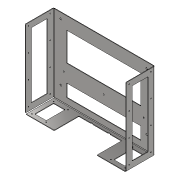
# Autodesk Inventor part: Display_Mount_B
Saved by Autodesk Inventor 2020 (Build 240168000, 168)
## iProperties
Created: 2021-12-05
Part Number: Display_Mount_B
Material: ステンレス鋼
Document SubType Name: Sheet Metal
Designer: ken113
Density: 8 g/cm^3
Sheet Metal Rule: Default_mm
Appearance: 半つや出し
Mass: 1681.3 g
Surface Area: 2199.78 cm^2
Volume: 210.162 cm^3
Author: ken113
Autodesk Inventor part; units mm, degrees
ref_plane "YZ Plane" through (0, 0, 0) normal (1, 0, 0) x (0, 1, 0)
ref_plane "XZ Plane" through (0, 0, 0) normal (0, 1, 0) x (-1, 0, 0)
ref_plane "XY Plane" through (0, 0, 0) normal (0, 0, 1) x (1, 0, 0)
sketch "スケッチ1" plane through (0, 0, 0) normal (0, 0, 1) x (1, 0, 0)
  line L0 (173, -134) -> (-173, -134)
  line L1 (-173, -134) -> (-173, 134)
  line L2 (-173, 134) -> (173, 134)
  line L3 (173, 134) -> (173, -134)
  line L4 (173, -134) -> (-173, 134) construction
  line L5 (-173, -134) -> (173, 134) construction
  point P0 (0, 0)
  dimension "d0" = 268
  dimension "d1" = 346
  measures "d0" distance of L0.end L1.end
  measures "d1" distance of L1.end L2.end
extrude "プレート1" add sketch "スケッチ1" along normal blind 2
sketch "スケッチ2" plane through (173, -136, 4) normal (0, -1, 0) x (1, 0, 0)
  line L0 (-346, 0) -> (0, 0)
  line L1 (0, 0) -> (0, 96)
  line L2 (0, 96) -> (-346, 96)
  line L3 (-346, 96) -> (-346, 0)
  constraints: 6 end point, 1 horizontal, 1 perpendicular, 1 vertical
edge flange "フランジ1" height 100 angle 90 thickness 2 bend radius 2 thickness toward (0, -1, 0) relief straight relief width 2 relief depth 1 edges at (0, -134, 2) wall of the first edge with corners at (-173, -136, 4) (173, -136, 4) (173, -136, 100) (-173, -136, 100)
bend "曲げ1"
corner "コーナー1"
sketch "スケッチ3" plane through (0, 0, 2) normal (0, 0, 1) x (1, 0, 0)
  line L0 (150, -86) -> (-150, -86)
  line L1 (-150, -86) -> (-150, 114)
  line L2 (-150, 114) -> (150, 114)
  line L3 (150, 114) -> (150, -86)
  line L4 (150, -86) -> (-150, 114) construction
  line L5 (-150, -86) -> (150, 114) construction
  line L6 (173, -134) -> (-173, -134) projected
  line L7 (-173, 134) -> (173, 134) projected
  point P0 (0, 0)
  point P1 (0, 14)
  point P2 (0, 14)
  dimension "d13" = 300
  dimension "d14" = 200
  dimension "d51" = 120
  constraints: 12 end point, 3 midpoint, 2 parallel, 1 horizontal, 1 perpendicular, 1 vertical alignment
  measures "d13" distance of L0.start L0.end
  measures "d14" distance of L0.end L1.end
  measures "d51" distance from line of L7 point (0, 14)
hole "穴1" at (-150, 114, 2) at (-150, -86, 2) at (150, -86, 2) at (150, 114, 2) direction (0, 0, -1) diameter 6.2 depth 2 tip angle 118
sketch "スケッチ4" plane through (0, 0, 2) normal (0, 0, 1) x (1, 0, 0)
  line L0 (130, -9.8) -> (-130, -9.8)
  line L1 (-130, -9.8) -> (-130, 90.2)
  line L2 (-130, 90.2) -> (130, 90.2)
  line L3 (130, 90.2) -> (130, -9.8)
  line L4 (130, -9.8) -> (-130, 90.2) construction
  line L5 (-130, -9.8) -> (130, 90.2) construction
  circle A0 centre (-150, 114) radius 3.1 projected
  point P0 (0, 0)
  point P1 (0, 40.2)
  point P2 (0, 40.2)
  dimension "d23" = 100
  dimension "d24" = 23.8
  dimension "d25" = 260
  constraints: 12 end point, 3 midpoint, 2 parallel, 1 horizontal, 1 perpendicular, 1 vertical alignment
  measures "d23" distance of L2.end L0.start
  measures "d24" distance from line of L2 A0.centre
  measures "d25" distance of L1.end L2.end
extrude "押し出し1" cut sketch "スケッチ4" against normal through all contours L0 L1 L2 L3
fillet "フィレット1" radius 2 4 edges at (130, -9.8, 1) (130, 90.2, 1) (-130, 90.2, 1) (-130, -9.8, 1)
sketch "スケッチ6" plane through (175, 134, 4) normal (1, 0, 0) x (0, 1, 0)
  line L0 (-268, 0) -> (0, 0)
  line L1 (0, 0) -> (0, 96)
  line L2 (0, 96) -> (-268, 96)
  line L3 (-268, 96) -> (-268, 0)
  constraints: 6 end point, 1 horizontal, 1 perpendicular, 1 vertical
edge flange "フランジ2" height 100 angle 90 thickness 2 bend radius 2 thickness toward (1, 0, 0) relief straight relief width 2 relief depth 1 corner gap 2 corner form 0 edges at (173, 0, 2) (-173, 0, 2) wall of the first edge with corners at (175, -134, 4) (175, 134, 4) (175, 134, 100) (175, -134, 100)
bend "曲げ2"
corner "コーナー2"
fillet "フィレット2" radius 2 6 edges at (-176, 134, 100) (-176, -134, 100) (-173, -137, 100) (173, -137, 100) (176, -134, 100) (176, 134, 100)
sketch "スケッチ7" plane through (-177, -134, 4) normal (-1, 0, 0) x (0, 0, 1)
  arc A0 (94, 0) -> (96, 2) centre (94, 2) ccw projected
  line L0 (96, 266) -> (96, 2) projected
  arc A1 (96, 266) -> (94, 268) centre (94, 266) ccw projected
  line L1 (0, 268) -> (94, 268) projected
  line L2 (0, 268) -> (0, 0) projected
  line L3 (94, 0) -> (0, 0) projected
  line L4 (10, 258) -> (86, 258)
  line L5 (86, 258) -> (86, 14)
  line L6 (86, 14) -> (10, 14)
  line L7 (10, 14) -> (10, 258)
  line L8 (10, 95.3333) -> (86, 95.3333)
  line L9 (86, 95.3333) -> (86, 176.6667)
  line L10 (86, 176.6667) -> (10, 176.6667)
  line L11 (10, 176.6667) -> (10, 95.3333)
  point P0 (-4, 134)
  dimension "d52" = 10
  dimension "d53" = 10
  dimension "d54" = 10
  dimension "d55" = 14
  dimension "d56" = 244
  dimension "d57" = 81.3333
  dimension "d58" = 81.3333
  constraints: 16 end point, 4 parallel, 2 horizontal, 2 perpendicular, 2 point on line
  measures "d52" distance between parallel lines of L7 L2
  measures "d53" distance between parallel lines of L1 L4
  measures "d54" distance between parallel lines of L0 L5
  measures "d55" distance between parallel lines of L6 L3
  measures "d56" distance of L4.end L5.end
  measures "d57" distance between parallel lines of L4 L10
  measures "d58" distance between parallel lines of L10 L8
hole "穴3" at (-177, -120, 14) at (-177, -120, 90) at (-177, -38.6667, 90) at (-177, -38.6667, 14) at (-177, 42.6667, 14) at (-177, 42.6667, 90) at (-177, 124, 90) at (-177, 124, 14) direction (1, 0, 0) diameter 3.242 end through all thread size "M4x0.7" class "6H" standard "ISO Metric profile"
sketch "スケッチ8" plane through (-173, -138, 4) normal (0, -1, 0) x (1, 0, 0)
  arc A0 (346, 94) -> (344, 96) centre (344, 94) ccw projected
  line L0 (2, 96) -> (344, 96) projected
  arc A1 (2, 96) -> (0, 94) centre (2, 94) ccw projected
  line L1 (0, 0) -> (0, 94) projected
  line L2 (0, 0) -> (346, 0) projected
  line L3 (346, 94) -> (346, 0) projected
  line L4 (10, 86) -> (60, 86)
  line L5 (60, 86) -> (60, 10)
  line L6 (60, 10) -> (10, 10)
  line L7 (10, 10) -> (10, 86)
  line L8 (286, 10) -> (336, 10)
  line L9 (336, 10) -> (336, 86)
  line L10 (336, 86) -> (286, 86)
  line L11 (286, 86) -> (286, 10)
  point P0 (173, -4)
  dimension "d66" = 50
  dimension "d67" = 50
  dimension "d68" = 10
  dimension "d69" = 10
  dimension "d70" = 10
  dimension "d71" = 10
  constraints: 16 end point, 4 parallel, 2 horizontal, 2 horizontal alignment, 2 perpendicular, 1 point on line
  measures "d66" distance of L4.start L4.end
  measures "d67" distance of L9.end L10.end
  measures "d68" distance between parallel lines of L6 L2
  measures "d69" distance between parallel lines of L0 L10
  measures "d70" distance between parallel lines of L3 L9
  measures "d71" distance between parallel lines of L1 L7
hole "穴4" at (-163, -138, 14) at (-113, -138, 90) at (-113, -138, 14) at (-163, -138, 90) at (113, -138, 14) at (163, -138, 14) at (163, -138, 90) at (113, -138, 90) direction (0, 1, 0) diameter 3.242 end through all thread size "M4x0.7" class "6H" standard "ISO Metric profile"
sketch "スケッチ9" plane through (-177, -134, 4) normal (-1, 0, 0) x (0, 0, 1)
  circle A0 centre (86, 258) radius 1.621 projected
  circle A1 centre (10, 176.6667) radius 1.621 projected
  circle A2 centre (86, 95.3333) radius 1.621 projected
  circle A3 centre (10, 14) radius 1.621 projected
  circle A4 centre (86, 14) radius 1.621 projected
  circle A5 centre (10, 95.3333) radius 1.621 projected
  circle A6 centre (86, 176.6667) radius 1.621 projected
  circle A7 centre (10, 258) radius 1.621 projected
  arc A8 (94, 0) -> (96, 2) centre (94, 2) ccw projected
  line L0 (96, 266) -> (96, 2) projected
  arc A9 (96, 266) -> (94, 268) centre (94, 266) ccw projected
  line L1 (0, 268) -> (94, 268) projected
  line L2 (0, 268) -> (0, 0) projected
  line L3 (94, 0) -> (0, 0) projected
  line L4 (20, 248) -> (76, 248)
  line L5 (76, 248) -> (76, 20)
  line L6 (76, 20) -> (20, 20)
  line L7 (20, 20) -> (20, 248)
  point P0 (-4, 134)
  dimension "d79" = 20
  dimension "d80" = 20
  dimension "d81" = 20
  dimension "d82" = 20
  constraints: 8 end point, 2 parallel, 1 horizontal, 1 perpendicular
  measures "d79" distance between parallel lines of L0 L5
  measures "d80" distance between parallel lines of L2 L7
  measures "d81" distance between parallel lines of L1 L4
  measures "d82" distance between parallel lines of L3 L6
extrude "押し出し2" cut sketch "スケッチ9" against normal through all contours L4 L5 L6 L7
fillet "フィレット3" radius 2 8 edges at (-176, 114, 24) (-176, 114, 80) (-176, -114, 24) (-176, -114, 80) (176, -114, 24) (176, -114, 80) (176, 114, 80) (176, 114, 24)
sketch "スケッチ11" plane through (0, 0, 2) normal (0, 0, 1) x (1, 0, 0)
  line L0 (130, 88.2) -> (130, -7.8) projected
  arc A0 (128, -9.8) -> (130, -7.8) centre (128, -7.8) ccw projected
  line L1 (128, -9.8) -> (-128, -9.8) projected
  arc A1 (-130, -7.8) -> (-128, -9.8) centre (-128, -7.8) ccw projected
  line L2 (-130, -7.8) -> (-130, 88.2) projected
  arc A2 (-128, 90.2) -> (-130, 88.2) centre (-128, 88.2) ccw projected
  line L3 (-128, 90.2) -> (128, 90.2) projected
  arc A3 (130, 88.2) -> (128, 90.2) centre (128, 88.2) ccw projected
  circle A4 centre (150, -86) radius 3.1 projected
  circle A5 centre (-150, 114) radius 3.1 projected
  circle A6 centre (-150, -86) radius 3.1 projected
  circle A7 centre (150, 114) radius 3.1 projected
  line L4 (-173, -134) -> (-173, 134) projected
  line L5 (173, -134) -> (-173, -134) projected
  line L6 (173, 134) -> (173, -134) projected
  line L7 (-173, 134) -> (173, 134) projected
  point P0 (0, 0)
  point P1 (-140, -39.8)
  point P2 (0, -39.8)
  point P3 (140, -39.8)
  dimension "d89" = 140
  dimension "d94" = 30
  constraints: 1 horizontal, 1 vertical alignment, 2 other
  measures "d89" distance of point (-140, -39.8) point (0, -39.8)
  measures "d94" distance from line of L1 point (-140, -39.8)
hole "穴5" at (-140, -39.8, 2) at (0, -39.8, 2) at (140, -39.8, 2) direction (0, 0, -1) diameter 4.3 end through all
sketch "スケッチ12" plane through (0, 0, 0) normal (0, 0, -1) x (-1, 0, 0)
  circle A0 centre (0, -39.8) radius 2.15 projected
  circle A1 centre (140, -39.8) radius 2.15 projected
  circle A2 centre (-140, -39.8) radius 2.15 projected
  line L0 (-130, -7.8) -> (-130, 88.2) projected
  arc A3 (-128, 90.2) -> (-130, 88.2) centre (-128, 88.2) ccw projected
  line L1 (-128, 90.2) -> (128, 90.2) projected
  arc A4 (130, 88.2) -> (128, 90.2) centre (128, 88.2) ccw projected
  line L2 (130, 88.2) -> (130, -7.8) projected
  arc A5 (128, -9.8) -> (130, -7.8) centre (128, -7.8) ccw projected
  line L3 (128, -9.8) -> (-128, -9.8) projected
  arc A6 (-130, -7.8) -> (-128, -9.8) centre (-128, -7.8) ccw projected
  circle A7 centre (-150, -86) radius 3.1 projected
  circle A8 centre (150, 114) radius 3.1 projected
  circle A9 centre (150, -86) radius 3.1 projected
  circle A10 centre (-150, 114) radius 3.1 projected
  line L4 (-173, -134) -> (173, -134) projected
  line L5 (173, -134) -> (173, 134) projected
  line L6 (173, 134) -> (-173, 134) projected
  line L7 (-173, 134) -> (-173, -134) projected
  point P0 (0, 0)
hole "穴6" at (140, -39.8, 0) at (0, -39.8, 0) at (-140, -39.8, 0) direction (0, 0, 1) diameter 4.2 end through all countersink diameter 8 countersink angle 90
sketch "スケッチ13" plane through (0, 0, 2) normal (0, 0, 1) x (1, 0, 0)
  line L0 (-130, -114) -> (130, -114)
  line L1 (130, -114) -> (130, -69.8)
  line L2 (130, -69.8) -> (-130, -69.8)
  line L3 (-130, -69.8) -> (-130, -114)
  circle A0 centre (0, -39.8) radius 2.15 projected
  line L4 (173, -134) -> (-173, -134) projected
  point P0 (0, 0)
  point P1 (-130, 88.2)
  point P2 (130, -7.8)
  dimension "d109" = 30
  dimension "d110" = 20
  constraints: 8 end point, 2 parallel, 2 vertical alignment, 1 horizontal, 1 perpendicular
  measures "d109" distance from line of A0.centre L2
  measures "d110" distance between parallel lines of L0 L4
extrude "押し出し3" cut sketch "スケッチ13" against normal blind 10 contours L3 L2 L1 L0
fillet "フィレット4" radius 2 4 edges at (-130, -69.8, 1) (-130, -114, 1) (130, -114, 1) (130, -69.8, 1)
sketch "スケッチ14" plane through (-173, -136, 4) normal (0, 1, 0) x (1, 0, 0)
  line L0 (2, -96) -> (344, -96) projected
  line L1 (98, -96) -> (248, -96)
  line L2 (248, -96) -> (248, -10)
  line L3 (248, -10) -> (98, -10)
  line L4 (98, -10) -> (98, -96)
  line L5 (0, 2) -> (346, 2) projected
  line L6 (346, 0) -> (0, 0) projected
  point P0 (173, 4)
  point P1 (173, 4)
  dimension "d114" = 150
  dimension "d115" = 75
  dimension "d120" = 10
  constraints: 8 end point, 2 parallel, 1 coincident, 1 horizontal, 1 perpendicular, 1 point on line
  measures "d114" distance between parallel lines of L2 L4
  measures "d115" distance from line of L2 point (173, 4)
  measures "d120" distance between parallel lines of L3 L6
extrude "押し出し4" cut sketch "スケッチ14" against normal blind 10
fillet "フィレット5" radius 2 4 edges at (-75, -137, 100) (-75, -137, 14) (75, -137, 100) (75, -137, 14)
sketch "スケッチ15" plane through (-173, -138, 4) normal (0, -1, 0) x (1, 0, 0)
  line L0 (246, 10) -> (100, 10) projected
  point P0 (173, -4)
  point P1 (143, 14)
  point P2 (203, 14)
  dimension "d122" = 60
  dimension "d123" = 30
  dimension "d131" = 4
  constraints: 1 horizontal alignment
  measures "d122" distance of point (143, 14) point (203, 14)
  measures "d123" horizontal distance of point (203, 14) point (173, -4)
  measures "d131" distance from line of L0 point (143, 14)
hole "穴7" at (-30, -138, 18) at (30, -138, 18) direction (0, 1, 0) diameter 12 end through all
sketch "スケッチ16" plane through (-173, -136, 4) normal (0, 1, 0) x (1, 0, 0)
  arc A0 (147.4721, -10) -> (138.5279, -10) centre (143, -14) ccw projected
  line L0 (147.4721, -10) -> (198.5279, -10) projected
  arc A1 (207.4721, -10) -> (198.5279, -10) centre (203, -14) ccw projected
  line L1 (207.4721, -10) -> (246, -10) projected
  arc A2 (248, -12) -> (246, -10) centre (246, -12) ccw projected
  line L2 (248, -12) -> (248, -94) projected
  arc A3 (248, -94) -> (250, -96) centre (250, -94) ccw projected
  line L3 (250, -96) -> (344, -96) projected
  arc A4 (344, -96) -> (346, -94) centre (344, -94) ccw projected
  line L4 (346, -94) -> (346, 0) projected
  line L5 (346, 0) -> (0, 0) projected
  line L6 (0, -94) -> (0, 0) projected
  arc A5 (0, -94) -> (2, -96) centre (2, -94) ccw projected
  line L7 (2, -96) -> (96, -96) projected
  arc A6 (96, -96) -> (98, -94) centre (96, -94) ccw projected
  line L8 (98, -94) -> (98, -12) projected
  arc A7 (100, -10) -> (98, -12) centre (100, -12) ccw projected
  line L9 (100, -10) -> (138.5279, -10) projected
  circle A8 centre (336, -86) radius 1.621 projected
  circle A9 centre (286, -10) radius 1.621 projected
  circle A10 centre (60, -10) radius 1.621 projected
  circle A11 centre (10, -10) radius 1.621 projected
  circle A12 centre (60, -86) radius 1.621 projected
  circle A13 centre (10, -86) radius 1.621 projected
  circle A14 centre (336, -10) radius 1.621 projected
  circle A15 centre (286, -86) radius 1.621 projected
  circle A16 centre (10, -10) radius 1.621 projected
  circle A17 centre (60, -86) radius 1.621 projected
  line L10 (10, -10) -> (60, -10)
  line L11 (60, -10) -> (60, -86)
  line L12 (60, -86) -> (10, -86)
  line L13 (10, -86) -> (10, -10)
  circle A18 centre (286, -10) radius 1.621 projected
  circle A19 centre (336, -86) radius 1.621 projected
  line L14 (286, -10) -> (336, -10)
  line L15 (336, -10) -> (336, -86)
  line L16 (336, -86) -> (286, -86)
  line L17 (286, -86) -> (286, -10)
  line L18 (55, -15) -> (15, -15)
  line L19 (15, -15) -> (15, -81)
  line L20 (15, -81) -> (55, -81)
  line L21 (55, -81) -> (55, -15)
  line L22 (331, -15) -> (291, -15)
  line L23 (291, -15) -> (291, -81)
  line L24 (291, -81) -> (331, -81)
  line L25 (331, -81) -> (331, -15)
  point P0 (173, 4)
  dimension "d132" = 5
  dimension "d133" = 5
  constraints: 32 end point, 8 parallel, 4 perpendicular, 2 horizontal, 6 other
  measures "d132" distance between parallel lines of L11 L21
  measures "d133" distance between parallel lines of L17 L23
extrude "押し出し5" cut sketch "スケッチ16" against normal blind 10 contours L21 L20 L19 L18 | L25 L24 L23 L22
fillet "フィレット6" radius 2 8 edges at (-118, -137, 85) (-158, -137, 85) (-158, -137, 19) (-118, -137, 19) (118, -137, 85) (118, -137, 19) (158, -137, 85) (158, -137, 19)
equation "\"d21\" = Thickness"
equation "\"d57\" = 0.333333 * d56"
equation "\"d58\" = d57"
equation "\"d129\" = Thickness"
equation "\"d2\" = Thickness"
equation "\"d3\" = BendReliefWidth"
equation "\"d4\" = BendReliefDepth"
equation "\"d5\" = MinimumRemnant"
equation "\"d6\" = TransitionRadius"
equation "\"d9\" = BendRadius"
equation "\"d10\" = CornerReliefSize"
equation "\"d11\" = GapSize"
equation "\"d12\" = JacobiRadiusSize"
equation "\"d40\" = BendReliefWidth"
equation "\"d41\" = BendReliefDepth"
equation "\"d42\" = MinimumRemnant"
equation "\"d43\" = TransitionRadius"
equation "\"d46\" = BendRadius"
equation "\"d47\" = CornerReliefSize"
equation "\"d48\" = GapSize"
equation "\"d49\" = JacobiRadiusSize"
equation "\"BendRadius\" = Thickness"
equation "\"BendReliefWidth\" = Thickness"
equation "\"BendReliefDepth\" = 0.5 * Thickness"
equation "\"CornerReliefSize\" = 4 * Thickness"
equation "\"MinimumRemnant\" = 2 * Thickness"
equation "\"TransitionRadius\" = BendRadius"
equation "\"JacobiRadiusSize\" = BendRadius"
equation "\"GapSize\" = Thickness"
equation "\"Thickness\" = 2"
